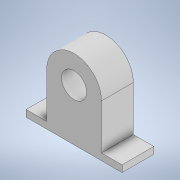
# Autodesk Inventor part: sopoetellantas
Saved by Autodesk Inventor 2021 (Build 250183000, 183)
## iProperties
Created: 2021-02-06
Part Number: sopoetellantas
Material: Genérico
Document SubType Name: Modeling
Designer: jaime
Density: 1 g/cm^3
Appearance: Valor por defecto
Author: jaime
Autodesk Inventor part; units mm, degrees
ref_plane "YZ Plane" through (0, 0, 0) normal (1, 0, 0) x (0, 1, 0)
ref_plane "XZ Plane" through (0, 0, 0) normal (0, 1, 0) x (-1, 0, 0)
ref_plane "XY Plane" through (0, 0, 0) normal (0, 0, 1) x (1, 0, 0)
sketch "Boceto1" plane through (0, 0, 0) normal (0, 0, 1) x (1, 0, 0)
  arc A0 (0, 8.616) -> (-8.616, 0) centre (0, 0) ccw
  line L0 (-8.616, 0) -> (-8.616, -14.1749)
  line L1 (-8.616, -14.1749) -> (-15.0769, -14.1749)
  line L2 (-15.0769, -14.1749) -> (-15.0769, -16.3011)
  line L3 (-15.0769, -16.3011) -> (0, -16.3011)
  line L4 (0, -16.3011) -> (0, 8.616) construction
  arc A1 (0, 3.9445) -> (0, -3.9445) centre (0, 0) ccw
  arc A2 (8.616, 0) -> (0, 8.616) centre (0, 0) ccw
  line L5 (8.616, 0) -> (8.616, -14.1749)
  line L6 (8.616, -14.1749) -> (15.0769, -14.1749)
  line L7 (15.0769, -14.1749) -> (15.0769, -16.3011)
  line L8 (15.0769, -16.3011) -> (0, -16.3011)
  arc A3 (0, -3.9445) -> (0, 3.9445) centre (0, 0) ccw
  constraints: 18 end point, 8 point on circle, 4 centre point, 4 symmetric about line, 3 coincident, 3 vertical, 2 point on line, 1 horizontal, 1 perpendicular, 1 tangent, 2 other
extrude "Extrusión1" add sketch "Boceto1" along normal blind 10
